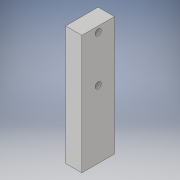
# Autodesk Inventor part: GlyphtMotorBrace
Saved by Autodesk Inventor 2017 (Build 210142000, 142)
## iProperties
Created: 2018-01-10
Part Number: GlyphtMotorBrace
Material: Generic
Document SubType Name: Modeling
Designer: User
Density: 1 g/cm^3
Appearance: Default
Author: User
Autodesk Inventor part; units mm, degrees
ref_plane "YZ Plane" through (0, 0, 0) normal (1, 0, 0) x (0, 1, 0)
ref_plane "XZ Plane" through (0, 0, 0) normal (0, 1, 0) x (-1, 0, 0)
ref_plane "XY Plane" through (0, 0, 0) normal (0, 0, 1) x (1, 0, 0)
sketch "Sketch1" plane through (0, 0, 0) normal (1, 0, 0) x (0, 1, 0)
  line L0 (0, 0) -> (69.85, 0)
  line L1 (69.85, 0) -> (69.85, -19.05)
  line L2 (69.85, -19.05) -> (0, -19.05)
  line L3 (0, -19.05) -> (0, 0)
  dimension "d0" = 19.05
  dimension "d1" = 69.85
  constraints: 8 end point, 2 parallel, 1 horizontal, 1 perpendicular
  measures "d0" distance of L0.end L1.end
  measures "d1" distance of L1.end L2.end
extrude "Extrusion1" add sketch "Sketch1" along normal blind 9.525
sketch "Sketch2" plane through (9.525, 0, 0) normal (1, 0, 0) x (0, 0, -1)
  line L0 (0, 69.85) -> (0, 0) projected
  line L1 (0, 0) -> (19.05, 0) projected
  line L2 (19.05, 0) -> (19.05, 69.85) projected
  line L3 (19.05, 69.85) -> (0, 69.85) projected
  point P0 (9.525, 66.675)
  point P1 (9.525, 39.7256)
  dimension "d4" = 26.9494
  dimension "d5" = 19.05
  dimension "d6" = 69.85
  dimension "d7" = 3.175
  dimension "d8" = 9.525
  dimension "d9" = 9.525
  measures "d4" distance of point (9.525, 39.726) point (9.525, 66.675)
  measures "d5" distance of L2.end L0.start
  measures "d6" distance of L0.start L0.end
  measures "d7" distance from line of L3 point (9.525, 66.675)
  measures "d8" distance from line of L0 point (9.525, 66.675)
  measures "d9" distance from line of L0 point (9.525, 39.726)
hole "Hole1" at (9.525, 66.675, -9.525) at (9.525, 39.7256, -9.525) direction (-1, 0, 0) diameter 3.556 depth 25.4 tip angle 118
sketch "Sketch3" plane through (0, 0, -19.05) normal (0, -1, 0) x (1, 0, 0)
  line L0 (0, 7.747) -> (9.525, 7.747) projected
  line L1 (0, 0) -> (0, 19.05) projected
  line L2 (0, 0) -> (9.525, 0) projected
  line L3 (9.525, 19.05) -> (9.525, 0) projected
  line L4 (0, 19.05) -> (9.525, 19.05) projected
  point P0 (4.7625, 15.875)
  point P1 (4.7625, 3.175)
  dimension "d17" = 19.05
  dimension "d18" = 9.525
  dimension "d19" = 4.7625
  dimension "d20" = 4.7625
  dimension "d21" = 12.7
  dimension "d22" = 3.175
  measures "d17" distance of L3.start L2.end
  measures "d18" distance of L1.end L3.start
  measures "d19" distance from line of L3 point (4.762, 15.875)
  measures "d20" distance from line of L3 point (4.763, 3.175)
  measures "d21" distance of point (4.762, 15.875) point (4.763, 3.175)
  measures "d22" distance from line of L2 point (4.763, 3.175)
hole "Hole2" at (4.7625, 0, -3.175) at (4.7625, 0, -15.875) direction (0, 1, 0) diameter 2.6416 depth 12.7 tip angle 118 thread size "6-32 UNC" class "2B" standard "ANSI Unified Screw Threads"
equation "\"d8\" = 0.5 * d5"
equation "\"d9\" = d8"
equation "\"d19\" = 0.5 * d18"
equation "\"d20\" = d19"
equation "\"d22\" = -0.5 * d21 + 0.5 * d17"
body "Solid1"
